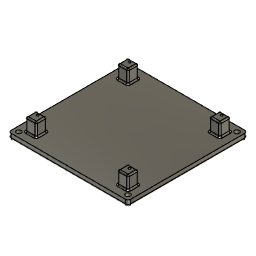
BuzzerBottom (Autodesk Fusion 360 design; units mm, degrees)
Autodesk Fusion 360 part; units mm, degrees
sketch "Sketch15" plane through (0, 0, 0) normal (0, 0, 1) x (1, 0, 0)
  line L0 (45.45, 45.45) -> (-45.45, 45.45)
  line L1 (-45.45, 45.45) -> (-45.45, -45.45)
  line L2 (-45.45, -45.45) -> (45.45, -45.45)
  line L3 (45.45, -45.45) -> (45.45, 45.45)
  dimension "d68" = 90.9
  dimension "d69" = 90.9
  constraint horizontal L0
  constraint perpendicular L0 L1
  constraint parallel L0 L2
  constraint parallel L1 L3
  measures "d68" distance of L1.end L2.end
  measures "d69" distance of L0.end L1.end
extrude "Extrude9" add sketch "Sketch15" along normal blind 5
sketch "Sketch16" plane through (0, 0, 5) normal (0, 0, 1) x (-1, 0, 0)
  line L0 (-45.45, 45.45) -> (-45.45, -45.45)
  line L1 (-45.45, -45.45) -> (45.45, -45.45)
  line L2 (45.45, -45.45) -> (45.45, 45.45)
  line L3 (45.45, 45.45) -> (-45.45, 45.45)
  line L4 (-39.45, -39.45) -> (39.45, -39.45)
  line L5 (39.45, -39.45) -> (39.45, 39.45)
  line L6 (39.45, 39.45) -> (-39.45, 39.45)
  line L7 (-39.45, 39.45) -> (-39.45, -39.45)
  line L8 (-39.45, -39.45) -> (39.45, 39.45) construction
  line L9 (39.45, -39.45) -> (-39.45, 39.45) construction
  line L10 (39.45, -39.45) -> (30.95, -39.45)
  line L11 (30.95, -39.45) -> (30.95, -30.95)
  line L12 (30.95, -30.95) -> (39.45, -30.95)
  line L13 (39.45, -30.95) -> (39.45, -39.45)
  line L14 (-39.45, -39.45) -> (-30.95, -39.45)
  line L15 (-30.95, -39.45) -> (-30.95, -30.95)
  line L16 (-30.95, -30.95) -> (-39.45, -30.95)
  line L17 (-39.45, -30.95) -> (-39.45, -39.45)
  line L18 (39.45, 39.45) -> (30.95, 39.45)
  line L19 (30.95, 39.45) -> (30.95, 30.95)
  line L20 (30.95, 30.95) -> (39.45, 30.95)
  line L21 (39.45, 30.95) -> (39.45, 39.45)
  line L22 (-39.45, 39.45) -> (-30.95, 39.45)
  line L23 (-30.95, 39.45) -> (-30.95, 30.95)
  line L24 (-30.95, 30.95) -> (-39.45, 30.95)
  line L25 (-39.45, 30.95) -> (-39.45, 39.45)
  line L26 (30.95, -30.95) -> (38.95, -30.95)
  line L27 (38.95, -30.95) -> (38.95, -38.95)
  line L28 (38.95, -38.95) -> (30.95, -38.95)
  line L29 (30.95, -38.95) -> (30.95, -30.95)
  line L30 (-30.95, -30.95) -> (-38.95, -30.95)
  line L31 (-38.95, -30.95) -> (-38.95, -38.95)
  line L32 (-38.95, -38.95) -> (-30.95, -38.95)
  line L33 (-30.95, -38.95) -> (-30.95, -30.95)
  line L34 (30.95, 30.95) -> (38.95, 30.95)
  line L35 (38.95, 30.95) -> (38.95, 38.95)
  line L36 (38.95, 38.95) -> (30.95, 38.95)
  line L37 (30.95, 38.95) -> (30.95, 30.95)
  line L38 (-30.95, 30.95) -> (-38.95, 30.95)
  line L39 (-38.95, 30.95) -> (-38.95, 38.95)
  line L40 (-38.95, 38.95) -> (-30.95, 38.95)
  line L41 (-30.95, 38.95) -> (-30.95, 30.95)
  dimension "d72" = 78.9
  dimension "d73" = 78.9
  dimension "d74" = 8.5
  dimension "d75" = 8.5
  dimension "d76" = 8.5
  dimension "d77" = 8.5
  dimension "d78" = 8.5
  dimension "d79" = 8.5
  dimension "d80" = 8.5
  dimension "d81" = 8.5
  dimension "d82" = 8
  dimension "d83" = 8
  dimension "d84" = 8
  dimension "d85" = 8
  dimension "d86" = 8
  dimension "d87" = 8
  dimension "d88" = 8
  dimension "d89" = 8
  constraint horizontal L4
  constraint perpendicular L4 L5
  constraint parallel L4 L6
  constraint parallel L5 L7
  constraint coincident L8 origin
  constraint coincident L9 origin
  constraint horizontal L10
  constraint vertical L11
  constraint horizontal L12
  constraint vertical L13
  constraint horizontal L14
  constraint vertical L15
  constraint horizontal L16
  constraint vertical L17
  constraint horizontal L18
  constraint vertical L19
  constraint horizontal L20
  constraint vertical L21
  constraint horizontal L22
  constraint vertical L23
  constraint horizontal L24
  constraint vertical L25
  constraint horizontal L26
  constraint vertical L27
  constraint horizontal L28
  constraint vertical L29
  constraint horizontal L30
  constraint vertical L31
  constraint horizontal L32
  constraint vertical L33
  constraint horizontal L34
  constraint vertical L35
  constraint horizontal L36
  constraint vertical L37
  constraint horizontal L38
  constraint vertical L39
  constraint horizontal L40
  constraint vertical L41
  measures "d72" distance of L5.end L6.end
  measures "d73" distance of L4.end L5.end
  measures "d74" distance of L4.end L10.end
  measures "d75" distance of L4.end L12.end
  measures "d76" distance of L4.start L14.end
  measures "d77" distance of L4.start L16.end
  measures "d78" distance of L5.end L18.end
  measures "d79" distance of L5.end L20.end
  measures "d80" distance of L6.end L22.end
  measures "d81" distance of L6.end L24.end
  measures "d82" distance of L11.end L26.end
  measures "d83" distance of L11.end L28.end
  measures "d84" distance of L15.end L30.end
  measures "d85" distance of L15.end L32.end
  measures "d86" distance of L19.end L34.end
  measures "d87" distance of L19.end L36.end
  measures "d88" distance of L23.end L38.end
  measures "d89" distance of L23.end L40.end
extrude "Extrude10" add sketch "Sketch16" along normal blind 10 contours L15 L16 L30 L31 L32 L33 | L11 L12 L26 L27 L28 L29 | L23 L24 L38 L39 L40 L41 | L19 L20 L34 L35 L36 L37
sketch "Sketch17" plane through (0, 0, 15) normal (0, 0, 1) x (-1, 0, 0)
  line L0 (39.4192, -39.4543) -> (35.3192, -39.4543)
  line L1 (39.4192, -36.5543) -> (39.4192, -39.4543)
  circle A0 centre (35.3192, -36.5543) radius 0.85
  circle A1 centre (-34.6808, -36.5543) radius 0.85
  line L2 (-34.6808, -35.7043) -> (-34.6808, 32.5957)
  line L3 (34.4692, -36.5543) -> (-33.8308, -36.5543)
  circle A2 centre (-34.6808, 33.4457) radius 0.85
  circle A3 centre (35.3192, 33.4457) radius 0.85
  line L4 (35.3192, -35.7043) -> (35.3192, 32.5957)
  line L5 (-33.8308, 33.4457) -> (34.4692, 33.4457)
  line L6 (-30.95, -38.95) -> (-30.95, -30.95)
  line L7 (-30.95, -30.95) -> (-38.95, -30.95)
  line L8 (-38.95, -30.95) -> (-38.95, -38.95)
  line L9 (-38.95, -38.95) -> (-30.95, -38.95)
  dimension "d92" = 4.1
  dimension "d93" = 2.9
  dimension "d94" = 1.7
  dimension "d95" = 70
  dimension "d96" = 70
  dimension "d97" = 1.7
  dimension "d98" = 70
  dimension "d99" = 1.7
  dimension "d101" = 1.7
  constraint horizontal L0
  constraint vertical L1
  constraint coincident A0 L3.start
  constraint coincident A0 L4.start
  constraint coincident A1 L3.end
  constraint coincident A1 L2.start
  constraint coincident A2 L2.end
  constraint coincident A2 L5.start
  constraint coincident A3 L4.end
  constraint coincident A3 L5.end
  constraint perpendicular L2 L5
  measures "d92" distance of L0.start L0.end
  measures "d93" distance of L0.start L1.start
  measures "d94" diameter of A0
  measures "d95" distance of A0.centre A1.centre
  measures "d96" distance of A0.centre A3.centre
  measures "d97" diameter of A1
  measures "d98" distance of A1.centre A2.centre
  measures "d99" diameter of A2
  measures "d101" diameter of A3
extrude "Extrude11" cut sketch "Sketch17" against normal blind 11 contours A0 | A3 | A1 | A2
sketch "Sketch18" plane through (0, 0, 5) normal (0, 0, 1) x (-1, 0, 0)
  line L0 (-45.5, -45.5) -> (-41.5, -45.5)
  line L1 (-41.5, -45.5) -> (-41.5, -43.3)
  line L2 (-43.3, -41.5) -> (-45.5, -41.5)
  line L3 (-45.5, -41.5) -> (-45.5, -45.5)
  circle A0 centre (-41.5, -41.5) radius 1.8
  line L4 (45.5, -45.5) -> (41.5, -45.5)
  line L5 (41.5, -45.5) -> (41.5, -43.3)
  line L6 (43.3, -41.5) -> (45.5, -41.5)
  line L7 (45.5, -41.5) -> (45.5, -45.5)
  circle A1 centre (41.5, -41.5) radius 1.8
  line L8 (45.5, 45.5) -> (41.5, 45.5)
  line L9 (41.5, 45.5) -> (41.5, 43.3)
  line L10 (43.3, 41.5) -> (45.5, 41.5)
  line L11 (45.5, 41.5) -> (45.5, 45.5)
  circle A2 centre (41.5, 41.5) radius 1.8
  line L12 (-45.5, 45.5) -> (-41.5, 45.5)
  line L13 (-45.5, 41.5) -> (-45.5, 45.5)
  circle A3 centre (-41.5, 41.5) radius 1.8
  line L14 (-41.5, 45.5) -> (-41.5, 43.3)
  line L15 (-43.3, 41.5) -> (-45.5, 41.5)
  dimension "d104" = 4
  dimension "d105" = 4
  dimension "d106" = 3.6
  dimension "d107" = 4
  dimension "d108" = 4
  dimension "d109" = 3.6
  dimension "d110" = 4
  dimension "d111" = 4
  dimension "d112" = 3.6
  dimension "d113" = 4
  dimension "d114" = 4
  dimension "d115" = 3.6
  constraint horizontal L0
  constraint vertical L1
  constraint horizontal L2
  constraint vertical L3
  constraint coincident A0 L2.start
  constraint coincident A0 L1.end
  constraint horizontal L4
  constraint vertical L5
  constraint horizontal L6
  constraint vertical L7
  constraint coincident A1 L6.start
  constraint coincident A1 L5.end
  constraint horizontal L8
  constraint vertical L9
  constraint horizontal L10
  constraint vertical L11
  constraint coincident A2 L9.end
  constraint coincident A2 L10.start
  constraint horizontal L12
  constraint vertical L13
  constraint coincident A3 L14.end
  constraint vertical L14
  constraint coincident A3 L15.start
  constraint horizontal L15
  measures "d104" distance of L0.start L0.end
  measures "d105" distance of L0.start L2.end
  measures "d106" diameter of A0
  measures "d107" distance of L4.start L4.end
  measures "d108" distance of L4.start L6.end
  measures "d109" diameter of A1
  measures "d110" distance of L8.start L8.end
  measures "d111" distance of L8.start L10.end
  measures "d112" diameter of A2
  measures "d113" distance of L12.start L12.end
  measures "d114" distance of L12.start L13.start
  measures "d115" diameter of A3
extrude "Extrude12" cut sketch "Sketch18" against normal blind 5 contours A0 | A1 | A2 | A3
fillet "Fillet4" radius 1 12 edges at (30.95, 34.95, 15) (34.95, 30.95, 15) (38.95, 34.95, 15) (34.95, 38.95, 15) (34.95, 38.95, 5) (30.95, 34.95, 5) (38.95, 38.95, 10) (30.95, 38.95, 10) (30.95, 30.95, 10) (34.95, 30.95, 5) (38.95, 30.95, 10) (38.95, 34.95, 5)
fillet "Fillet5" radius 1 12 edges at (-30.95, 34.95, 15) (-34.95, 30.95, 15) (-38.95, 34.95, 15) (-34.95, 38.95, 15) (-30.95, 38.95, 10) (-30.95, 30.95, 10) (-30.95, 34.95, 5) (-34.95, 30.95, 5) (-38.95, 30.95, 10) (-38.95, 38.95, 10) (-34.95, 38.95, 5) (-38.95, 34.95, 5)
fillet "Fillet6" radius 1 12 edges at (38.95, -38.95, 10) (34.95, -38.95, 5) (38.95, -34.95, 5) (38.95, -30.95, 10) (38.95, -34.95, 15) (34.95, -38.95, 15) (30.95, -38.95, 10) (30.95, -34.95, 15) (34.95, -30.95, 15) (30.95, -30.95, 10) (34.95, -30.95, 5) (30.95, -34.95, 5)
fillet "Fillet7" radius 1 12 edges at (-38.95, -30.95, 10) (-38.95, -34.95, 15) (-34.95, -30.95, 15) (-30.95, -30.95, 10) (-34.95, -30.95, 5) (-38.95, -34.95, 5) (-38.95, -38.95, 10) (-34.95, -38.95, 15) (-30.95, -34.95, 15) (-30.95, -38.95, 10) (-34.95, -38.95, 5) (-30.95, -34.95, 5)
fillet "Fillet8" radius 2 4 edges at (0, -45.45, 0) (45.45, 0, 0) (0, 45.45, 0) (-45.45, 0, 0)
fillet "Fillet9" radius 2 8 edges at (44.8642, -44.8642, 0.5858) (45.45, -45.45, 3.5) (-44.8642, -44.8642, 0.5858) (-45.45, -45.45, 3.5) (44.8642, 44.8642, 0.5858) (45.45, 45.45, 3.5) (-44.8642, 44.8642, 0.5858) (-45.45, 45.45, 3.5)
